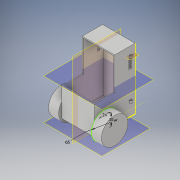
# Autodesk Inventor part: Pieza1
Saved by Autodesk Inventor 2018 (Build 220112000, 112)
## iProperties
Created: 2019-02-10
Part Number: Pieza1
Material: Genérico
Document SubType Name: Modeling
Designer: EDWIN
Density: 1 g/cm^3
Appearance: Valor por defecto
Author: EDWIN
Autodesk Inventor part; units mm, degrees
ref_plane "YZ Plane" through (0, 0, 0) normal (1, 0, 0) x (0, 1, 0)
ref_plane "XZ Plane" through (0, 0, 0) normal (0, 1, 0) x (-1, 0, 0)
ref_plane "XY Plane" through (0, 0, 0) normal (0, 0, 1) x (1, 0, 0)
sketch "Boceto1" plane through (0, 0, 0) normal (0, 0, 1) x (1, 0, 0)
  line L0 (-40, 75) -> (40, 75)
  line L1 (40, 75) -> (40, -75)
  line L2 (40, -75) -> (-40, -75)
  line L3 (-40, -75) -> (-40, 75)
  line L4 (-40, 75) -> (40, -75) construction
  line L5 (40, 75) -> (-40, -75) construction
  line L6 (37.5, 72.5) -> (-37.5, 72.5)
  line L7 (-37.5, 72.5) -> (-37.5, -74.5)
  line L8 (-37.5, -74.5) -> (37.5, -74.5)
  line L9 (37.5, -74.5) -> (37.5, 72.5)
  point P0 (0, 0)
  dimension "d0" = 80
  dimension "d1" = 150
  dimension "d2" = 2.5
  dimension "d32" = 0.5
  constraints: 20 end point, 3 parallel, 3 perpendicular, 2 midpoint, 1 horizontal, 1 other
  measures "d0" distance of L1.end L2.end
  measures "d1" distance of L0.end L1.end
  measures "d2" distance between parallel lines of L0 L6
  measures "d32" distance between parallel lines of L8 L2
extrude "Extrusión1" add sketch "Boceto1" along normal blind 50
extrude "Extrusión2" add sketch "Boceto1" along normal blind 0.5 contours L9 L8 L7 L6
sketch "Boceto2" plane through (40, -75, 0) normal (1, 0, 0) x (0, 0, -1)
  circle A0 centre (-75, 14.3207) radius 32.5
  line L0 (-106.2586, 14.1414) -> (-42.2586, 14.1414) construction
  line L1 (0, 0) -> (-50, 0) projected
  line L2 (-87, 2.3207) -> (-63, 2.3207)
  line L3 (-63, 2.3207) -> (-63, 32.3207)
  line L4 (-63, 32.3207) -> (-87, 32.3207)
  line L5 (-87, 32.3207) -> (-87, 2.3207)
  line L6 (-0.5, 0.5) -> (-50, 0.5) projected
  line L7 (0, 150) -> (0, 0) projected
  line L8 (-49.75, 14.1414) -> (25.25, 14.1414) construction
  point P0 (0, 75)
  dimension "d9" = 65
  dimension "d15" = 24
  dimension "d16" = 30
  constraints: 12 end point, 3 horizontal, 2 parallel, 1 centre point, 1 perpendicular
  measures "d9" diameter of A0
  measures "d15" distance of L4.end L3.end
  measures "d16" distance of L3.end L2.end
extrude "Extrusión3" cut sketch "Boceto2" against normal blind 10 contours L5 L4 L3 L2
extrude "Extrusión4" add sketch "Boceto2" along normal blind 25 contours A0 | L5 L4 L3 L2
mirror "Simetría1" about plane through (0, 0, 0) normal (1, 0, 0) of "Extrusión4", "Extrusión3"
sketch "Boceto3" plane through (40, -75, 0) normal (0, -1, 0) x (1, 0, 0)
  line L0 (-80, 0) -> (-80, 50) projected
  line L1 (-2.5, 0.5) -> (-2.5, 50) projected
  line L2 (-80, 107.5) -> (-80, 45.8252) projected
  line L3 (-80, 50) -> (-80, 100)
  line L4 (-80, 100) -> (0, 100)
  line L5 (0, 0) -> (0, 50) projected
  line L6 (0, 100) -> (0, 50)
  line L7 (0, 50) -> (-2.5, 50)
  line L8 (-2.5, 50) -> (-2.5, 97.5)
  line L9 (-2.5, 97.5) -> (-77.5, 97.5)
  line L10 (-77.5, 97.5) -> (-77.5, 50)
  line L11 (-77.5, 50) -> (-80, 50)
  line L12 (-77.5, 50) -> (-2.5, 50) projected
  line L13 (-77.5, 50) -> (-2.5, 50)
  point P0 (-40, 0)
  dimension "d24" = 50
  dimension "d25" = 80
  dimension "d26" = 47.5
  dimension "d27" = 75
  constraints: 18 end point, 3 perpendicular, 1 collinear, 1 horizontal, 1 vertical
  measures "d24" distance of L0.end L3.end
  measures "d25" distance of L3.end L4.end
  measures "d26" distance of L1.end L8.end
  measures "d27" distance of L8.end L9.end
extrude "Extrusión5" add sketch "Boceto3" against normal blind 70 contours L4 L6 L7 L8 L9 L10 L11 L2
extrude "Extrusión6" add sketch "Boceto3" against normal blind 0.5 contours L10 L9 L8 L12
extrude "Extrusión7" cut sketch "Boceto2" against normal blind 80 contours L5 L4 L3 L2
ref_plane "Plano de trabajo1" through (-40, -93.1793, 75) normal (0, -1, 0) x (1, 0, 0)
sketch "Boceto4" plane through (40, -75, 0) normal (1, 0, 0) x (0, 0, -1)
  line L0 (0, 0) -> (0, 150) projected
  line L1 (21.5, -18.1793) -> (-129, -18.1793) projected
  line L2 (-12, 31.3207) -> (-12, 131.3207) construction
  line L3 (-21.5167, 81.3207) -> (7.9238, 81.3207)
  line L4 (-0.5, 147.5) -> (-0.5, 0.5) projected
  line L5 (-8, 131.3207) -> (-8, 121.3207)
  line L6 (-8.9804, 121.3207) -> (-14.9804, 121.3207)
  line L7 (-14.9804, 121.3207) -> (-14.9804, 101.3207)
  line L8 (-14.9804, 101.3207) -> (-8.9804, 101.3207)
  line L9 (-8.9804, 101.3207) -> (-8.9804, 121.3207)
  line L10 (-11, 101.3207) -> (-11, 103.5079)
  point P0 (0, 75)
  dimension "d39" = 100
  dimension "d45" = 24
  dimension "d46" = 10
  dimension "d47" = 8
  dimension "d49" = 20
  dimension "d53" = 6
  constraints: 16 end point, 4 parallel, 3 perpendicular, 1 horizontal, 1 point on line, 1 vertical
  measures "d39" distance of L2.start L2.end
  measures "d45" diameter of L0 L2
  measures "d46" distance of L5.end L5.start
  measures "d47" diameter of L5 L2
  measures "d49" distance of L7.end L6.end
  measures "d53" distance of L7.end L8.end
ref_plane "Plano de trabajo2" through (40, 56.3207, 12) normal (0, 1, 0) x (-1, 0, 0)
sketch "Boceto5" plane through (40, 56.3207, 12) normal (0, 1, 0) x (-1, 0, 0)
  line L0 (0, 0) -> (-2, 0)
  circle A0 centre (-2, 0) radius 2
  arc A1 (0, 2.2361) -> (0, -2.2361) centre (-2, 0) ccw
  line L1 (0, -2.2361) -> (0, 2.2361)
  point P0 (40, -12)
  dimension "d40" = 2
  dimension "d41" = 6
  constraints: 4 end point, 2 coincident, 2 point on circle, 1 centre point, 1 horizontal, 1 horizontal alignment, 1 vertical, 2 other
  measures "d40" distance of L0.start L0.end
  measures "d41" diameter of A1
extrude "Extrusión8" add sketch "Boceto5" against normal blind 5
ref_plane "Plano de trabajo3" through (40, 6.3207, 21.5167) normal (0, -1, 0) x (0, 0, -1)
mirror "Simetría2" about plane through (40, 6.3207, 21.5167) normal (0, -1, 0) of "Extrusión8"
extrude "Extrusión9" cut sketch "Boceto4" against normal through all
ref_plane "Plano de trabajo4" through (0, -75, 0) normal (1, 0, 0) x (0, 0, -1)
mirror "Simetría3" about plane through (0, -75, 0) normal (1, 0, 0) of "Extrusión8", "Simetría2"
